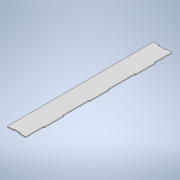
# Autodesk Inventor part: стенка 1
Saved by Autodesk Inventor 2021 (Build 250183000, 183)
## iProperties
Created: 2023-02-14
Part Number: стенка 1
Material: Типовые
Document SubType Name: Modeling
Designer: Tasya
Density: 1 g/cm^3
Appearance: По умолчанию
Author: Tasya
Autodesk Inventor part; units mm, degrees
ref_plane "YZ Plane" through (0, 0, 0) normal (1, 0, 0) x (0, 1, 0)
ref_plane "XZ Plane" through (0, 0, 0) normal (0, 1, 0) x (-1, 0, 0)
ref_plane "XY Plane" through (0, 0, 0) normal (0, 0, 1) x (1, 0, 0)
sketch "Эскиз1" plane through (0, 0, 0) normal (0, 1, 0) x (-1, 0, 0)
  line L0 (-42.5, 340.5) -> (42.5, 340.5)
  line L1 (42.5, 340.5) -> (42.5, -340.5)
  line L2 (42.5, -340.5) -> (-42.5, -340.5)
  line L3 (-42.5, -340.5) -> (-42.5, 340.5)
  line L4 (-42.5, 340.5) -> (42.5, -340.5) construction
  line L5 (42.5, 340.5) -> (-42.5, -340.5) construction
  line L6 (-42.5, 258.5) -> (-42.5, 168.5)
  line L7 (-42.5, 168.5) -> (-46.5, 168.5)
  line L8 (-46.5, 168.5) -> (-46.5, 258.5)
  line L9 (-46.5, 258.5) -> (-42.5, 258.5)
  line L10 (0, 0) -> (-44.5, 0) construction
  line L11 (-42.5, -258.5) -> (-42.5, -168.5)
  line L12 (-42.5, -168.5) -> (-46.5, -168.5)
  line L13 (-46.5, -168.5) -> (-46.5, -258.5)
  line L14 (-46.5, -258.5) -> (-42.5, -258.5)
  line L15 (-42.5, 45) -> (-46.5, 45)
  line L16 (-46.5, 45) -> (-46.5, -45)
  line L17 (-46.5, -45) -> (-42.5, -45)
  line L18 (-42.5, -45) -> (-42.5, 45)
  line L19 (-42.5, 45) -> (-46.5, -45) construction
  line L20 (-46.5, 45) -> (-42.5, -45) construction
  line L21 (-15, 336.5) -> (15, 336.5)
  line L22 (15, 336.5) -> (15, 340.5)
  line L23 (15, 340.5) -> (-15, 340.5)
  line L24 (-15, 340.5) -> (-15, 336.5)
  line L25 (-15, 336.5) -> (15, 340.5) construction
  line L26 (15, 336.5) -> (-15, 340.5) construction
  line L27 (0, 47.7496) -> (0, 0) construction
  line L28 (-15, -336.5) -> (15, -336.5)
  line L29 (15, -336.5) -> (15, -340.5)
  line L30 (15, -340.5) -> (-15, -340.5)
  line L31 (-15, -340.5) -> (-15, -336.5)
  point P0 (-42.5, -168.5)
  point P1 (-42.5, -258.5)
  point P2 (-44.5, 0)
  point P3 (-42.5, -45)
  point P4 (-42.5, 45)
  point P5 (0, 338.5)
  point P6 (-15, -340.5)
  point P7 (15, -340.5)
  dimension "d0" = 681
  dimension "d1" = 85
  dimension "d2" = 4
  dimension "d3" = 90
  dimension "d7" = 90
  dimension "d8" = 4
  dimension "d9" = 4
  dimension "d10" = 30
  dimension "d11" = 123.5
  constraints: 64 end point, 8 parallel, 8 symmetric about line, 7 midpoint, 4 horizontal, 4 perpendicular, 2 collinear, 2 point on line, 1 vertical, 1 other
  measures "d0" distance of L2.end L0.start
  measures "d1" distance between parallel lines of L3 L1
  measures "d2" distance of L6.end L7.end
  measures "d3" distance of L7.end L8.end
  measures "d7" distance of L15.end L16.end
  measures "d8" distance of L16.end L17.end
  measures "d9" distance of L23.end L21.start
  measures "d10" distance of L21.start L21.end
  measures "d11" distance between parallel lines of L15 L7
extrude "Выдавливание1" add sketch "Эскиз1" along normal blind 4 contours L0 L24 L21 L22 L1 L2 L29 L28 L31 L3 | L3 L7 L8 L9 | L3 L17 L16 L15 | L3 L14 L13 L12
